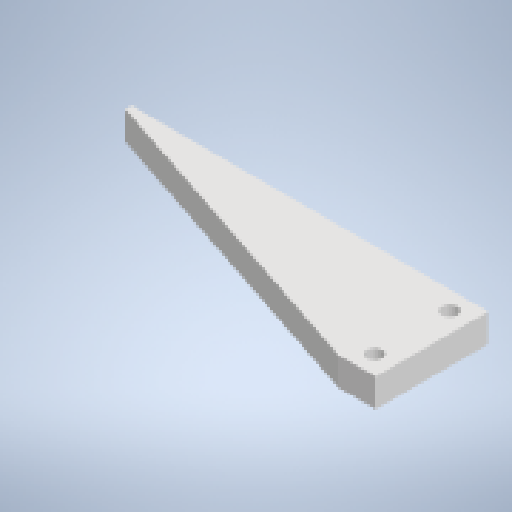
# Autodesk Inventor part: Gripper triangle
Saved by Autodesk Inventor 2023 (Build 270158000, 158)
## iProperties
Created: 2023-02-27
Part Number: Gripper triangle
Material: Generic
Document SubType Name: Modeling
Designer: Gabriel - T3 CAD
Density: 1 g/cm^3
Appearance: Default
Author: Gabriel - T3 CAD
Autodesk Inventor part; units mm, degrees
ref_plane "YZ Plane" through (0, 0, 0) normal (1, 0, 0) x (0, 1, 0)
ref_plane "XZ Plane" through (0, 0, 0) normal (0, 1, 0) x (-1, 0, 0)
ref_plane "XY Plane" through (0, 0, 0) normal (0, 0, 1) x (1, 0, 0)
sketch "Sketch1" plane through (0, 0, 0) normal (0, 1, 0) x (-1, 0, 0)
  line L0 (0, 0) -> (12.7, 0)
  line L1 (12.7, 0) -> (12.7, 50.8)
  line L2 (12.7, 50.8) -> (0, 50.8)
  line L3 (0, 50.8) -> (0, 0)
  circle A0 centre (6.8152, 44.45) radius 2.5797
  circle A1 centre (6.8152, 19.05) radius 2.5797
  line L4 (0, 0) -> (127, 0)
  line L5 (127, 0) -> (127, 12.7)
  line L6 (127, 12.7) -> (0, 12.7)
  line L7 (0, 12.7) -> (0, 0)
  line L8 (12.7, 50.8) -> (127, 12.7)
  line L9 (0, 12.7) -> (127, 12.7)
  line L10 (127, 12.7) -> (127, 11.1125)
  line L11 (127, 11.1125) -> (0, 11.1125)
  line L12 (0, 11.1125) -> (0, 12.7)
  line L13 (0, 12.7) -> (19.05, 12.7)
  line L14 (19.05, 12.7) -> (19.05, 11.1125)
  line L15 (19.05, 11.1125) -> (0, 11.1125)
  line L16 (0, 11.1125) -> (0, 12.7)
  line L17 (127, 12.7) -> (120.65, 12.7)
  line L18 (120.65, 12.7) -> (120.65, 11.1125)
  line L19 (120.65, 11.1125) -> (127, 11.1125)
  line L20 (127, 11.1125) -> (127, 12.7)
  line L21 (120.65, 12.7) -> (120.65, 14.8167)
  point P0 (120.65, 11.1125)
  point P1 (120.65, 12.7)
  point P2 (19.05, 12.7)
  point P3 (19.05, 11.1125)
  dimension "d0" = 12.7
  dimension "d1" = 6.8152
  dimension "d2" = 6.8152
  dimension "d3" = 25.4
  dimension "d4" = 19.05
  dimension "d5" = 6.35
  dimension "d6" = 5.1594
  dimension "d7" = 127
  dimension "d8" = 12.7
  dimension "d9" = 127
  dimension "d10" = 1.5875
  dimension "d15" = 19.05
  dimension "d16" = 1.5875
  dimension "d17" = 6.35
  dimension "d18" = 1.5875
  constraints: 44 end point, 10 parallel, 5 horizontal, 5 perpendicular, 2 centre point, 1 equal radius, 1 point on line, 1 vertical
  measures "d0" distance of L2.end L1.end
  measures "d1" distance from line of L3 A0.centre
  measures "d2" distance from line of L3 A1.centre
  measures "d3" distance of A1.centre A0.centre
  measures "d4" distance from line of L0 A1.centre
  measures "d5" distance from line of L2 A0.centre
  measures "d6" diameter of A0
  measures "d7" distance of L6.end L5.end
  measures "d8" distance of L5.end L4.end
  measures "d9" distance of L10.end L11.end
  measures "d10" distance of L9.end L10.end
  measures "d15" distance of L14.end L15.end
  measures "d16" distance of L13.end L14.end
  measures "d17" distance of L19.end L18.end
  measures "d18" distance of L18.end L17.end
extrude "Extrusion1" add sketch "Sketch1" along normal mid plane 9.525 contours L3 L2 L1 L6 | L1 L8 L21 L6
extrude "Extrusion2" add sketch "Sketch1" along normal mid plane 6.35 contours L14 L6 L18 L11
equation "\"d2\" = d1"
equation "\"d16\" = d18"
body "Solid1"
